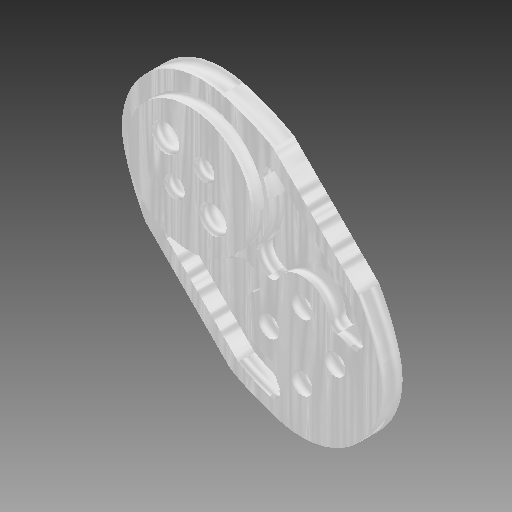
# Autodesk Inventor part: 脚クランクハッピーターン最終段1
Saved by Autodesk Inventor 2020 (Build 240168000, 168)
## iProperties
Created: 2019-07-23
Part Number: 脚クランクハッピーターン最終段1
Material: アルミニウム 7075
Document SubType Name: Modeling
Designer: 雪村
Density: 2.81 g/cm^3
Appearance: サテン - ブラシ仕上げ 重厚
Mass: 4.09217 g
Surface Area: 19.5249 cm^2
Volume: 1.45629 cm^3
Description: アルミ7000 4t
Author: 雪村
Autodesk Inventor part; units mm, degrees
ref_plane "YZ Plane" through (0, 0, 0) normal (1, 0, 0) x (0, 1, 0)
ref_plane "XZ Plane" through (0, 0, 0) normal (0, 1, 0) x (-1, 0, 0)
ref_plane "XY Plane" through (0, 0, 0) normal (0, 0, 1) x (1, 0, 0)
sketch "スケッチ1" plane through (0, 0, 0) normal (0, 0, 1) x (1, 0, 0)
  circle A0 centre (-12.0208, 12.0208) radius 9.55
  circle A1 centre (0, 0) radius 6
  arc A2 (-9.5747, 16.4536) -> (-16.4536, 9.5747) centre (-14.8669, 14.8669) ccw
  arc A3 (-7.588, 14.467) -> (-9.5747, 16.4536) centre (-10.253, 13.7886) ccw
  circle A4 centre (0, 0) radius 9.55
  arc A5 (9.2246, 2.4717) -> (-9.5491, 21.2454) centre (-16.4207, -4.3999) ccw
  arc A6 (-21.2454, 9.5491) -> (-2.4717, -9.2246) centre (4.3999, 16.4207) ccw
  circle A7 centre (-14.8669, 14.8669) radius 2
  circle A8 centre (-9.1747, 9.1747) radius 2
  circle A9 centre (-13.7886, 10.253) radius 1.25
  circle A10 centre (-10.253, 13.7886) radius 1.25
  line L0 (0, 3.9598) -> (3.9598, 0)
  line L1 (3.9598, 0) -> (0, -3.9598)
  line L2 (0, -3.9598) -> (-3.9598, 0)
  line L3 (-3.9598, 0) -> (0, 3.9598)
  line L4 (0, 0) -> (0, 3.9598)
  circle A11 centre (0, 0) radius 1.25
  circle A12 centre (0, 3.9598) radius 1.25
  circle A13 centre (3.9598, 0) radius 1.25
  circle A14 centre (0, -3.9598) radius 1.25
  circle A15 centre (-3.9598, 0) radius 1.25
  dimension "d4" = 12
  dimension "d5" = 19.1
  dimension "d6" = 26.55
  dimension "d7" = 26.55
  dimension "d8" = 5.6
  dimension "d9" = 2.5
  dimension "d10" = 2.5
  dimension "d11" = 2.5
  dimension "d12" = 2.5
  dimension "d13" = 2.5
  constraints: 16 centre point, 12 point on circle, 10 end point, 8 coincident, 4 tangent, 2 vertical, 18 other
  measures "d4" diameter of A1
  measures "d5" diameter of A4
  measures "d6" radius of A5
  measures "d7" radius of A6
  measures "d8" distance of L2.end L0.start
  measures "d9" diameter of A11
  measures "d10" diameter of A12
  measures "d11" diameter of A13
  measures "d12" diameter of A14
  measures "d13" diameter of A15
extrude "押し出し1" add sketch "スケッチ1" along normal blind 4 contours A0 A4 | A0 A5 A4 | A4 A0 | A0 A4 | A4 A6 A0 | A1 | L0 A13 L1 A14 L2 A15 L3 A12 | A11
sketch "スケッチ2" plane through (0, 0, 4) normal (0, 0, 1) x (1, 0, 0)
  circle A0 centre (-13.7886, 10.253) radius 1.25 projected
  arc A1 (-9.5491, 21.2454) -> (-21.2454, 9.5491) centre (-12.0208, 12.0208) ccw projected
  arc A2 (-21.2454, 9.5491) -> (-2.4717, -9.2246) centre (4.3999, 16.4207) ccw projected
  arc A3 (-2.4717, -9.2246) -> (9.2246, 2.4717) centre (0, 0) ccw projected
  arc A4 (9.2246, 2.4717) -> (-9.5491, 21.2454) centre (-16.4207, -4.3999) ccw projected
  circle A5 centre (-3.9598, 0) radius 1.25 projected
  circle A6 centre (0, -3.9598) radius 1.25 projected
  circle A7 centre (3.9598, 0) radius 1.25 projected
  circle A8 centre (0, 3.9598) radius 1.25 projected
  circle A9 centre (-14.8669, 14.8669) radius 2 projected
  circle A10 centre (-10.253, 13.7886) radius 1.25 projected
  circle A11 centre (-13.7886, 10.253) radius 1.25 projected
  circle A12 centre (-9.1747, 9.1747) radius 2 projected
  circle A13 centre (-12.0208, 12.0208) radius 7.5
  dimension "d17" = 15
  constraints: 1 centre point, 1 coincident
  measures "d17" diameter of A13
extrude "押し出し3" cut sketch "スケッチ2" against normal blind 1.5 contours A4 A3 A2 A1
sketch "スケッチ4" plane through (-12.0208, 12.0208, 4) normal (0, 0, 1) x (1, 0, 0)
  circle A0 centre (0, 0) radius 7.5 projected
  circle A1 centre (-2.8461, 2.8461) radius 2 projected
  circle A2 centre (1.7678, 1.7678) radius 1.25 projected
  circle A3 centre (-1.7678, -1.7678) radius 1.25 projected
  circle A4 centre (2.8461, -2.8461) radius 2 projected
  circle A5 centre (-2.8461, 2.8461) radius 1.65
  circle A6 centre (2.8461, -2.8461) radius 1.65
  point P0 (12.0208, -12.0208)
  dimension "d23" = 3.3
  dimension "d24" = 3.3
  constraints: 2 centre point, 2 coincident
  measures "d23" diameter of A5
  measures "d24" diameter of A6
extrude "押し出し4" add sketch "スケッチ4" against normal blind 4 contours A1 | A4
sketch "スケッチ6" plane through (0, 0, 2.5) normal (0, 0, 1) x (1, 0, 0)
  circle A0 centre (-9.1747, 9.1747) radius 1.65 projected
  circle A1 centre (-14.8669, 14.8669) radius 1.65 projected
  circle A2 centre (-12.0208, 12.0208) radius 7.5 projected
  circle A3 centre (-10.253, 13.7886) radius 1.25 projected
  circle A4 centre (-13.7886, 10.253) radius 1.25 projected
  arc A5 (-2.4717, -9.2246) -> (9.2246, 2.4717) centre (0, 0) ccw projected
  arc A6 (9.2246, 2.4717) -> (-9.5491, 21.2454) centre (-16.4207, -4.3999) ccw projected
  arc A7 (-9.5491, 21.2454) -> (-21.2454, 9.5491) centre (-12.0208, 12.0208) ccw projected
  arc A8 (-21.2454, 9.5491) -> (-2.4717, -9.2246) centre (4.3999, 16.4207) ccw projected
  circle A9 centre (3.9598, 0) radius 1.25 projected
  circle A10 centre (0, 3.9598) radius 1.25 projected
  circle A11 centre (-3.9598, 0) radius 1.25 projected
  circle A12 centre (0, -3.9598) radius 1.25 projected
  circle A13 centre (-12.0208, 12.0208) radius 7.5 projected
  line L0 (-26.6598, 11.3473) -> (-2.3521, -12.9604)
  line L1 (-7.0354, 22.3479) -> (13.1284, 2.1841)
  line L2 (0, 0) -> (-12.0208, 12.0208)
  point P0 (-3.4581, 18.7706)
  point P1 (6.7498, 8.5627)
  point P2 (-8.5627, -6.7498)
  point P3 (-18.7706, 3.4581)
  dimension "d28" = 1
  dimension "d29" = 1
  constraints: 6 end point, 2 parallel
  measures "d28" distance edge to line of A6 L1
  measures "d29" distance edge to line of A8 L0
extrude "押し出し5" cut sketch "スケッチ6" against normal through all contours A8 L0 | L1 A6
sketch "スケッチ7" plane through (0, 0, 2.5) normal (0, 0, 1) x (1, 0, 0)
  line L0 (6.7498, 8.5627) -> (-3.4581, 18.7706) projected
  arc A0 (-3.4581, 18.7706) -> (-9.5491, 21.2454) centre (-16.4207, -4.3999) ccw projected
  arc A1 (-9.5491, 21.2454) -> (-21.2454, 9.5491) centre (-12.0208, 12.0208) ccw projected
  arc A2 (-21.2454, 9.5491) -> (-18.7706, 3.4581) centre (4.3999, 16.4207) ccw projected
  line L1 (-18.7706, 3.4581) -> (-8.5627, -6.7498) projected
  arc A3 (-8.5627, -6.7498) -> (-2.4717, -9.2246) centre (4.3999, 16.4207) ccw projected
  arc A4 (-2.4717, -9.2246) -> (9.2246, 2.4717) centre (0, 0) ccw projected
  arc A5 (9.2246, 2.4717) -> (6.7498, 8.5627) centre (-16.4207, -4.3999) ccw projected
  circle A6 centre (3.9598, 0) radius 1.25 projected
  circle A7 centre (0, 3.9598) radius 1.25 projected
  circle A8 centre (-3.9598, 0) radius 1.25 projected
  circle A9 centre (0, -3.9598) radius 1.25 projected
  circle A10 centre (-12.0208, 12.0208) radius 7.5 projected
  circle A11 centre (-12.0208, 12.0208) radius 8
  line L2 (-7.6512, -5.54) -> (-17.5608, 4.3696)
  arc A12 (-19.7965, 9.9373) -> (-17.5608, 4.3696) centre (4.3999, 16.4207) ccw
  arc A13 (-9.9373, 19.7965) -> (-19.7965, 9.9373) centre (-12.0208, 12.0208) ccw
  arc A14 (-4.3696, 17.5608) -> (-9.9373, 19.7965) centre (-16.4207, -4.3999) ccw
  line L3 (-4.3696, 17.5608) -> (5.54, 7.6512)
  arc A15 (7.7757, 2.0835) -> (5.54, 7.6512) centre (-16.4207, -4.3999) ccw
  arc A16 (-2.0835, -7.7757) -> (7.7757, 2.0835) centre (0, 0) ccw
  arc A17 (-7.6512, -5.54) -> (-2.0835, -7.7757) centre (4.3999, 16.4207) ccw
  circle A18 centre (0, 3.9598) radius 3.25
  circle A19 centre (3.9598, 0) radius 3.25
  circle A20 centre (0, -3.9598) radius 3.25
  circle A21 centre (-3.9598, 0) radius 3.25
  circle A22 centre (-3.7187, 15.4956) radius 1
  circle A23 centre (6.2716, 3.5662) radius 1
  circle A24 centre (-3.5662, -6.2716) radius 1
  circle A25 centre (-15.4956, 3.7187) radius 1
  point P0 (-15.1095, 4.6411)
  point P1 (-16.2027, 3.0116)
  point P2 (-3.8975, -7.2152)
  point P3 (-2.7271, -5.7277)
  point P4 (-3.1466, -3.1466)
  point P5 (-3.1466, 3.1466)
  point P6 (3.1466, 3.1466)
  point P7 (5.7277, 2.7271)
  point P8 (7.2152, 3.8975)
  point P9 (-3.0116, 16.2027)
  point P10 (-4.6411, 15.1095)
  dimension "d32" = 0.5
  dimension "d33" = 1.5
  dimension "d34" = 2
  dimension "d35" = 2
  dimension "d36" = 2
  dimension "d37" = 2
  dimension "d38" = 2
  dimension "d39" = 2
  dimension "d40" = 2
  dimension "d41" = 2
  constraints: 15 centre point, 12 point on circle, 8 tangent, 4 end point, 7 other
  measures "d32" radial gap between concentric circles of A10 A11
  measures "d33" distance between parallel lines of L1 L2
  measures "d34" radial gap between concentric circles of A7 A18
  measures "d35" radial gap between concentric circles of A6 A19
  measures "d36" radial gap between concentric circles of A9 A20
  measures "d37" radial gap between concentric circles of A8 A21
  measures "d38" diameter of A22
  measures "d39" diameter of A23
  measures "d40" diameter of A24
  measures "d41" diameter of A25
extrude "押し出し6" cut sketch "スケッチ7" against normal through all contours A11 A22 L3 A15 A23 A19 A18 A21 A20 A24 A17 L2 A25 | A22 | A25 | A23 | A24
sketch "スケッチ8" plane through (0, 0, 2.5) normal (0, 0, 1) x (1, 0, 0)
  circle A0 centre (-9.1747, 9.1747) radius 1.65 projected
  circle A1 centre (-14.8669, 14.8669) radius 1.65 projected
  circle A2 centre (-12.0208, 12.0208) radius 7.5 projected
  circle A3 centre (-10.253, 13.7886) radius 1.25 projected
  circle A4 centre (-13.7886, 10.253) radius 1.25 projected
  line L0 (-12.0208, 12.0208) -> (0, 0)
  arc A5 (-15.1095, 4.6411) -> (-4.6411, 15.1095) centre (-12.0208, 12.0208) ccw projected
  arc A6 (-3.1466, 3.1466) -> (-3.1466, -3.1466) centre (-3.9598, 0) ccw projected
  arc A7 (3.1466, 3.1466) -> (-3.1466, 3.1466) centre (0, 3.9598) ccw projected
  arc A8 (-4.8837, 3.1159) -> (-7.3173, 5.5496) centre (-7.2313, 3.2019) ccw
  arc A9 (-5.5496, 7.3173) -> (-3.1159, 4.8837) centre (-3.2019, 7.2313) ccw
  line L1 (-3.9598, 0) -> (-1.9799, 1.9799)
  dimension "d44" = 0.5
  dimension "d45" = 0.5
  dimension "d46" = 1.25
  dimension "d47" = 1.25
  dimension "d48" = 1.25
  dimension "d49" = 1.25
  constraints: 8 point on circle, 4 end point, 2 centre point, 2 point on line
  measures "d44" distance edge to line of A9 L0
  measures "d45" distance edge to line of A8 L0
  measures "d46" distance from line of L0 A8.end
  measures "d47" distance from line of L0 A9.start
  measures "d48" distance from line of A8.start L0
  measures "d49" distance from line of L0 A9.end
extrude "押し出し7" add sketch "スケッチ8" against normal blind 2.5 contours A5 A9 A7 L0 | L0 A6 A8 A5
fillet "フィレット1" radius 1 6 edges at (-3.1466, -3.1466, 1.25) (-4.8837, 3.1159, 1.25) (-7.3173, 5.5496, 1.25) (-5.5496, 7.3173, 1.25) (-3.1159, 4.8837, 1.25) (3.1466, 3.1466, 1.25)
sketch "スケッチ9" plane through (0, 0, 0) normal (0, 0, -1) x (-1, 0, 0)
  arc A0 (7.5795, 5.3669) -> (15.1095, 4.6411) centre (12.0208, 12.0208) ccw projected
  arc A1 (16.2027, 3.0116) -> (15.1095, 4.6411) centre (15.4956, 3.7187) ccw projected
  line L0 (16.2027, 3.0116) -> (7.6512, -5.54) projected
  arc A2 (3.8975, -7.2152) -> (7.6512, -5.54) centre (-4.3999, 16.4207) ccw projected
  arc A3 (2.7271, -5.7277) -> (3.8975, -7.2152) centre (3.5662, -6.2716) ccw projected
  arc A4 (2.7271, -5.7277) -> (3.2429, -4.1746) centre (0, -3.9598) ccw projected
  arc A5 (4.1746, -3.2429) -> (3.2429, -4.1746) centre (4.2407, -4.2407) ccw projected
  arc A6 (4.1746, -3.2429) -> (5.5131, 2.8548) centre (3.9598, 0) ccw projected
  arc A7 (5.0719, 4.1269) -> (5.5131, 2.8548) centre (5.9911, 3.7331) ccw projected
  arc A8 (6.8709, 5.5233) -> (5.0719, 4.1269) centre (7.2313, 3.2019) ccw projected
  arc A9 (7.5795, 5.3669) -> (6.8709, 5.5233) centre (7.0243, 4.5352) ccw projected
  arc A10 (4.1269, 5.0719) -> (5.5233, 6.8709) centre (3.2019, 7.2313) ccw projected
  arc A11 (2.8548, 5.5131) -> (4.1269, 5.0719) centre (3.7331, 5.9911) ccw projected
  arc A12 (2.8548, 5.5131) -> (-3.2429, 4.1746) centre (0, 3.9598) ccw projected
  arc A13 (-4.1746, 3.2429) -> (-3.2429, 4.1746) centre (-4.2407, 4.2407) ccw projected
  arc A14 (-4.1746, 3.2429) -> (-5.7277, 2.7271) centre (-3.9598, 0) ccw projected
  arc A15 (-7.2152, 3.8975) -> (-5.7277, 2.7271) centre (-6.2716, 3.5662) ccw projected
  arc A16 (-5.54, 7.6512) -> (-7.2152, 3.8975) centre (16.4207, -4.3999) ccw projected
  line L1 (-5.54, 7.6512) -> (3.0116, 16.2027) projected
  arc A17 (4.6411, 15.1095) -> (3.0116, 16.2027) centre (3.7187, 15.4956) ccw projected
  arc A18 (4.6411, 15.1095) -> (5.3669, 7.5795) centre (12.0208, 12.0208) ccw projected
  arc A19 (5.5233, 6.8709) -> (5.3669, 7.5795) centre (4.5352, 7.0243) ccw projected
  circle A20 centre (13.7886, 10.253) radius 1.25 projected
  circle A21 centre (10.253, 13.7886) radius 1.25 projected
  circle A22 centre (0, 3.9598) radius 1.25 projected
  circle A23 centre (-3.9598, 0) radius 1.25 projected
  circle A24 centre (0, -3.9598) radius 1.25 projected
  circle A25 centre (3.9598, 0) radius 1.25 projected
  line L2 (3.4581, 18.7706) -> (-6.7498, 8.5627) projected
  arc A26 (-6.7498, 8.5627) -> (-9.2246, 2.4717) centre (16.4207, -4.3999) ccw projected
  arc A27 (-9.2246, 2.4717) -> (2.4717, -9.2246) centre (0, 0) ccw projected
  arc A28 (2.4717, -9.2246) -> (8.5627, -6.7498) centre (-4.3999, 16.4207) ccw projected
  line L3 (8.5627, -6.7498) -> (18.7706, 3.4581) projected
  arc A29 (18.7706, 3.4581) -> (21.2454, 9.5491) centre (-4.3999, 16.4207) ccw projected
  arc A30 (21.2454, 9.5491) -> (9.5491, 21.2454) centre (12.0208, 12.0208) ccw projected
  arc A31 (9.5491, 21.2454) -> (3.4581, 18.7706) centre (16.4207, -4.3999) ccw projected
  circle A32 centre (14.8669, 14.8669) radius 1.65 projected
  circle A33 centre (9.1747, 9.1747) radius 1.65 projected
extrude "押し出し8" add sketch "スケッチ9" against normal blind 0.5 contours A0 A1 L0 A2 A3 A4 A5 A6 A7 A8 A9 | A11 A12 A13 A14 A15 A16 L1 A17 A18 A19 A10
sketch "スケッチ10" plane through (0, 0, 0) normal (0, 0, -1) x (-1, 0, 0)
  circle A0 centre (13.7886, 10.253) radius 1.25 projected
  circle A1 centre (10.253, 13.7886) radius 1.25 projected
  point P0 (0, 0)
extrude "押し出し9" add sketch "スケッチ10" against normal blind 1
sketch "スケッチ11" plane through (-12.0208, 12.0208, 4) normal (0, 0, 1) x (1, 0, 0)
  circle A0 centre (2.8461, -2.8461) radius 1.65 projected
  circle A1 centre (-2.8461, 2.8461) radius 1.65 projected
  circle A2 centre (0, 0) radius 7.5 projected
  circle A3 centre (1.7678, 1.7678) radius 1.25 projected
  circle A4 centre (-1.7678, -1.7678) radius 1.25 projected
  arc A5 (17.7485, -9.2937) -> (19.236, -8.1234) centre (18.2924, -8.4546) ccw projected
  arc A6 (19.236, -8.1234) -> (17.5608, -4.3696) centre (-4.3999, -16.4207) ccw projected
  line L0 (9.0093, 4.1819) -> (17.5608, -4.3696) projected
  arc A7 (9.0093, 4.1819) -> (7.3797, 3.0887) centre (8.3022, 3.4748) ccw projected
  arc A8 (6.6539, -4.4413) -> (7.3797, 3.0887) centre (0, 0) ccw projected
  arc A9 (6.6539, -4.4413) -> (6.4975, -5.1499) centre (7.4857, -4.9965) ccw projected
  arc A10 (6.4975, -5.1499) -> (7.8939, -6.949) centre (8.8189, -4.7895) ccw projected
  arc A11 (7.8939, -6.949) -> (9.1661, -6.5077) centre (8.2877, -6.0297) ccw projected
  arc A12 (15.2637, -7.8462) -> (9.1661, -6.5077) centre (12.0208, -8.061) ccw projected
  arc A13 (15.2637, -7.8462) -> (16.1954, -8.7779) centre (16.2615, -7.7801) ccw projected
  arc A14 (17.7485, -9.2937) -> (16.1954, -8.7779) centre (15.9806, -12.0208) ccw projected
  arc A15 (6.949, -7.8939) -> (5.1499, -6.4975) centre (4.7895, -8.8189) ccw projected
  arc A16 (5.1499, -6.4975) -> (4.4413, -6.6539) centre (4.9965, -7.4857) ccw projected
  arc A17 (-3.0887, -7.3797) -> (4.4413, -6.6539) centre (0, 0) ccw projected
  arc A18 (-3.0887, -7.3797) -> (-4.1819, -9.0093) centre (-3.4748, -8.3022) ccw projected
  line L1 (4.3696, -17.5608) -> (-4.1819, -9.0093) projected
  arc A19 (4.3696, -17.5608) -> (8.1234, -19.236) centre (16.4207, 4.3999) ccw projected
  arc A20 (8.1234, -19.236) -> (9.2937, -17.7485) centre (8.4546, -18.2924) ccw projected
  arc A21 (8.7779, -16.1954) -> (9.2937, -17.7485) centre (12.0208, -15.9806) ccw projected
  arc A22 (8.7779, -16.1954) -> (7.8462, -15.2637) centre (7.7801, -16.2615) ccw projected
  arc A23 (6.5077, -9.1661) -> (7.8462, -15.2637) centre (8.061, -12.0208) ccw projected
  arc A24 (6.5077, -9.1661) -> (6.949, -7.8939) centre (6.0297, -8.2877) ccw projected
  circle A25 centre (12.0208, -8.061) radius 1.25 projected
  circle A26 centre (15.9806, -12.0208) radius 1.25 projected
  circle A27 centre (12.0208, -15.9806) radius 1.25 projected
  circle A28 centre (8.061, -12.0208) radius 1.25 projected
  line L2 (8.5627, 6.7498) -> (18.7706, -3.4581) projected
  arc A29 (21.2454, -9.5491) -> (18.7706, -3.4581) centre (-4.3999, -16.4207) ccw projected
  arc A30 (9.5491, -21.2454) -> (21.2454, -9.5491) centre (12.0208, -12.0208) ccw projected
  arc A31 (3.4581, -18.7706) -> (9.5491, -21.2454) centre (16.4207, 4.3999) ccw projected
  line L3 (3.4581, -18.7706) -> (-6.7498, -8.5627) projected
  arc A32 (-9.2246, -2.4717) -> (-6.7498, -8.5627) centre (16.4207, 4.3999) ccw projected
  arc A33 (2.4717, 9.2246) -> (-9.2246, -2.4717) centre (0, 0) ccw projected
  arc A34 (8.5627, 6.7498) -> (2.4717, 9.2246) centre (-4.3999, -16.4207) ccw projected
  circle A35 centre (-2.8461, 2.8461) radius 1.65 projected
  circle A36 centre (2.8461, -2.8461) radius 1.65 projected
sketch "スケッチ12" plane through (0, 0, 0) normal (0, 0, -1) x (-1, 0, 0)
  circle A0 centre (0, 0) radius 1.25
  dimension "d57" = 2.5
  constraints: 1 centre point, 1 coincident
  measures "d57" diameter of A0
extrude "押し出し10" cut sketch "スケッチ12" against normal blind 1
equation "\"d6\" = d14"
equation "\"d7\" = d14"
equation "\"d45\" = d44"
equation "\"d47\" = d46"
equation "\"d48\" = d46"
equation "\"d49\" = d47"
equation "\"d14\" = 26.55"
